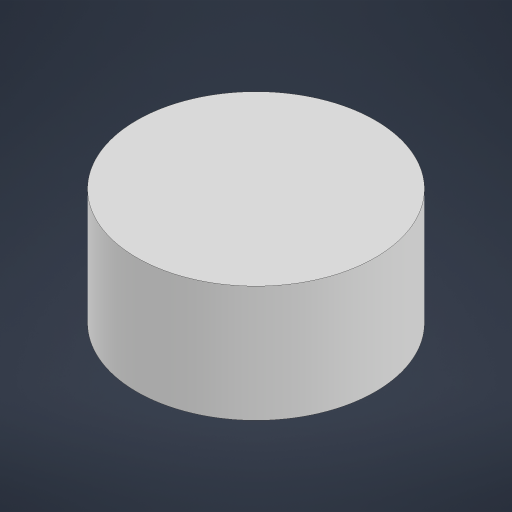
# Autodesk Inventor part: Test part
Saved by Autodesk Inventor 2024.1 (Build 281209000, 209)
## iProperties
Created: 2024-01-22
Part Number: Test part
Material: Generic
Document SubType Name: Modeling
Designer: vg3
Density: 1 g/cm^3
Appearance: Default
Author: vg3
Autodesk Inventor part; units mm, degrees
ref_plane "YZ Plane" through (0, 0, 0) normal (1, 0, 0) x (0, 1, 0)
ref_plane "XZ Plane" through (0, 0, 0) normal (0, 1, 0) x (-1, 0, 0)
ref_plane "XY Plane" through (0, 0, 0) normal (0, 0, 1) x (1, 0, 0)
sketch "Sketch1" plane through (0, 0, 0) normal (0, 1, 0) x (-1, 0, 0)
  circle A0 centre (4.6155, 11.5612) radius 26.0349
  point P0 (0, 0)
  dimension "d0" = 25.4
  constraints: 1 centre point
extrude "Extrusion1" add sketch "Sketch1" along normal blind 25.4
body "Solid1"
